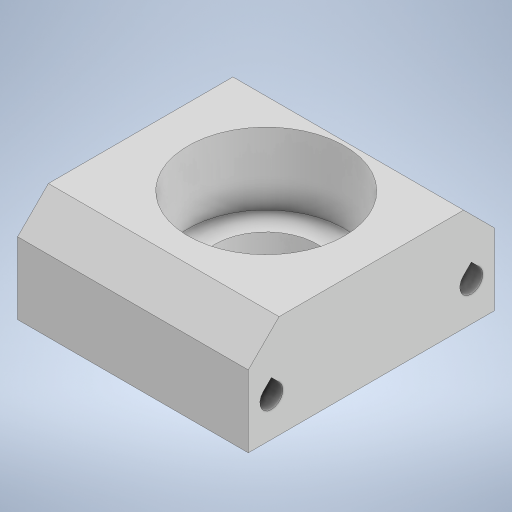
# Autodesk Inventor part: Część1-01
Saved by Autodesk Inventor 2023 (Build 270158000, 158)
## iProperties
Created: 2023-04-06
Part Number: Część1-01
Material: Ogólny
Document SubType Name: Modeling
Designer: Kamil
Density: 1 g/cm^3
Appearance: Domyślna
Author: Kamil
Autodesk Inventor part; units mm, degrees
ref_plane "YZ Plane" through (0, 0, 0) normal (1, 0, 0) x (0, 1, 0)
ref_plane "XZ Plane" through (0, 0, 0) normal (0, 1, 0) x (-1, 0, 0)
ref_plane "XY Plane" through (0, 0, 0) normal (0, 0, 1) x (1, 0, 0)
sketch "Szkic1" plane through (0, 0, 0) normal (0, 1, 0) x (-1, 0, 0)
  line L0 (22.5, 24) -> (-22.5, 24)
  line L1 (-22.5, 24) -> (-22.5, -24)
  line L2 (-22.5, -24) -> (22.5, -24)
  line L3 (22.5, -24) -> (22.5, 24)
  line L4 (22.5, 24) -> (-22.5, -24) construction
  line L5 (-22.5, 24) -> (22.5, -24) construction
  point P0 (0, 0)
  dimension "d0" = 45
  dimension "d1" = 48
  constraints: 12 end point, 2 midpoint, 2 parallel, 1 horizontal, 1 perpendicular
  measures "d0" distance of L2.end L1.end
  measures "d1" distance of L1.end L0.end
extrude "Wyciągnięcie proste1" add sketch "Szkic1" along normal blind 20
sketch "Szkic2" plane through (0, 20, 0) normal (0, 1, 0) x (1, 0, 0)
  line L0 (0, 0) -> (0, 2) construction
  dimension "d4" = 2
  constraints: 2 end point, 1 coincident, 1 vertical
  measures "d4" distance of L0.start L0.end
hole "Otwór1" at (0, 20, -2) direction (0, -1, 0) diameter 20 end through all counterbore diameter 30.5 counterbore depth 14
chamfer "Faza1" distance 6 angle 45 2 edges at (0, 20, -24) (0, 20, 24)
sketch "Szkic3" plane through (22.5, 0, 24) normal (1, 0, 0) x (0, 0, -1)
  line L0 (0, 0) -> (4.5, 0)
  line L1 (24, 0) -> (24, 9.8003)
  arc A0 (2.909, 8.891) -> (6.091, 8.891) centre (4.5, 7.3) ccw
  line L2 (4.5, 10.482) -> (6.091, 8.891)
  line L3 (4.5, 10.482) -> (2.909, 8.891)
  line L4 (0, 0) -> (48, 0) projected
  line L5 (0, 0) -> (0, 14) projected
  arc A1 (41.909, 8.891) -> (45.091, 8.891) centre (43.5, 7.3) ccw
  line L6 (43.5, 10.482) -> (41.909, 8.891)
  line L7 (43.5, 10.482) -> (45.091, 8.891)
  dimension "d17" = 4.5
  dimension "d20" = 7.3
  dimension "d21" = 4.5
  constraints: 12 end point, 4 point on circle, 4 symmetric about line, 2 centre point, 2 coincident, 1 horizontal, 1 tangent, 1 vertical, 1 other
  measures "d17" diameter of A0
  measures "d20" distance from line of L4 A0.centre
  measures "d21" distance from line of L5 A0.centre
extrude "Wyciągnięcie proste2" cut sketch "Szkic3" against normal through all
sketch "Szkic4" plane through (22.5, 0, -24) normal (0, 0, -1) x (-1, 0, 0)
  line L0 (12.305, 10.2206) -> (32.695, 10.2206) construction
  line L1 (32.695, 10.2206) -> (32.695, 3.7794) construction
  line L2 (32.695, 3.7794) -> (12.305, 3.7794) construction
  line L3 (12.305, 3.7794) -> (12.305, 10.2206) construction
  line L4 (22.5, -0.0035) -> (22.5, 22.4866) construction
  line L5 (0, 8.891) -> (45, 8.891) construction
  line L6 (0, 0) -> (0, 14) construction
  line L7 (17.4064, 4.002) -> (12.9229, 4.002)
  line L8 (12.9229, 4.002) -> (12.9229, 4.9956)
  spline S0 degree 2 poles (12.9229, 4.9956) (13.4914, 5.4503) (14.4009, 6.2511) (14.742, 6.612) knots 0 0 0 1 2 2 2
  spline S1 degree 2 poles (14.742, 6.612) (15.1919, 7.0816) (15.5923, 7.7984) (15.5923, 8.1741) knots 0 0 0 1 2 2 2
  spline S2 degree 2 poles (15.5923, 8.1741) (15.5923, 8.5992) (15.0831, 9.054) (14.6283, 9.054) knots 0 0 0 1 2 2 2
  spline S3 degree 2 poles (14.6283, 9.054) (14.396, 9.054) (13.9808, 8.9403) (13.7682, 8.8513) knots 0 0 0 1 2 2 2
  spline S4 degree 2 poles (13.7682, 8.8513) (13.5606, 8.7574) (13.264, 8.5597) (13.1898, 8.5102) knots 0 0 0 1 2 2 2
  line L9 (13.1898, 8.5102) -> (13.0712, 8.5102)
  line L10 (13.0712, 8.5102) -> (13.0712, 9.84)
  spline S5 degree 2 poles (13.0712, 9.84) (13.3282, 9.9635) (14.4257, 10.2206) (14.9348, 10.2206) knots 0 0 0 1 2 2 2
  spline S6 degree 2 poles (14.9348, 10.2206) (16.0223, 10.2206) (17.1395, 9.2517) (17.1395, 8.3768) knots 0 0 0 1 2 2 2
  spline S7 degree 2 poles (17.1395, 8.3768) (17.1395, 7.8379) (16.6304, 6.7999) (16.0421, 6.2067) knots 0 0 0 1 2 2 2
  spline S8 degree 2 poles (16.0421, 6.2067) (15.6714, 5.8409) (14.9744, 5.2724) (14.8211, 5.1537) knots 0 0 0 1 2 2 2
  line L11 (14.8211, 5.1537) -> (17.4064, 5.1537)
  line L12 (17.4064, 5.1537) -> (17.4064, 4.002)
  line L13 (23.6893, 4.002) -> (23.6893, 6.3006)
  spline S9 degree 2 poles (23.6893, 6.3006) (23.6893, 6.6417) (23.6646, 7.1063) (23.6053, 7.2546) knots 0 0 0 1 2 2 2
  spline S10 degree 2 poles (23.6053, 7.2546) (23.5411, 7.4029) (23.284, 7.5364) (23.0517, 7.5364) knots 0 0 0 1 2 2 2
  spline S11 degree 2 poles (23.0517, 7.5364) (22.8885, 7.5364) (22.5722, 7.393) (22.3843, 7.2596) knots 0 0 0 1 2 2 2
  line L14 (22.3843, 7.2596) -> (22.3843, 4.002)
  line L15 (22.3843, 4.002) -> (20.9409, 4.002)
  line L16 (20.9409, 4.002) -> (20.9409, 6.3006)
  spline S12 degree 2 poles (20.9409, 6.3006) (20.9409, 6.6367) (20.9112, 7.1063) (20.8519, 7.2546) knots 0 0 0 1 2 2 2
  spline S13 degree 2 poles (20.8519, 7.2546) (20.7876, 7.4029) (20.5306, 7.5364) (20.2983, 7.5364) knots 0 0 0 1 2 2 2
  spline S14 degree 2 poles (20.2983, 7.5364) (20.1252, 7.5364) (19.7842, 7.3733) (19.626, 7.2596) knots 0 0 0 1 2 2 2
  line L17 (19.626, 7.2596) -> (19.626, 4.002)
  line L18 (19.626, 4.002) -> (18.1924, 4.002)
  line L19 (18.1924, 4.002) -> (18.1924, 8.6041)
  line L20 (18.1924, 8.6041) -> (19.626, 8.6041)
  line L21 (19.626, 8.6041) -> (19.626, 8.095)
  spline S15 degree 2 poles (19.626, 8.095) (19.9769, 8.3916) (20.6047, 8.7277) (20.9953, 8.7277) knots 0 0 0 1 2 2 2
  spline S16 degree 2 poles (20.9953, 8.7277) (21.4154, 8.7277) (22.0581, 8.3273) (22.2261, 7.9269) knots 0 0 0 1 2 2 2
  spline S17 degree 2 poles (22.2261, 7.9269) (22.6364, 8.3125) (23.368, 8.7277) (23.7437, 8.7277) knots 0 0 0 1 2 2 2
  spline S18 degree 2 poles (23.7437, 8.7277) (24.065, 8.7277) (24.5742, 8.5251) (24.7472, 8.3174) knots 0 0 0 1 2 2 2
  spline S19 degree 2 poles (24.7472, 8.3174) (24.94, 8.095) (25.1328, 7.487) (25.1328, 6.9976) knots 0 0 0 1 2 2 2
  line L22 (25.1328, 6.9976) -> (25.1328, 4.002)
  line L23 (25.1328, 4.002) -> (23.6893, 4.002)
  line L24 (31.6876, 4.002) -> (31.6876, 6.3006)
  spline S20 degree 2 poles (31.6876, 6.3006) (31.6876, 6.6417) (31.6628, 7.1063) (31.6035, 7.2546) knots 0 0 0 1 2 2 2
  spline S21 degree 2 poles (31.6035, 7.2546) (31.5393, 7.4029) (31.2822, 7.5364) (31.0499, 7.5364) knots 0 0 0 1 2 2 2
  spline S22 degree 2 poles (31.0499, 7.5364) (30.8868, 7.5364) (30.5704, 7.393) (30.3825, 7.2596) knots 0 0 0 1 2 2 2
  line L25 (30.3825, 7.2596) -> (30.3825, 4.002)
  line L26 (30.3825, 4.002) -> (28.9391, 4.002)
  line L27 (28.9391, 4.002) -> (28.9391, 6.3006)
  spline S23 degree 2 poles (28.9391, 6.3006) (28.9391, 6.6367) (28.9094, 7.1063) (28.8501, 7.2546) knots 0 0 0 1 2 2 2
  spline S24 degree 2 poles (28.8501, 7.2546) (28.7859, 7.4029) (28.5288, 7.5364) (28.2965, 7.5364) knots 0 0 0 1 2 2 2
  spline S25 degree 2 poles (28.2965, 7.5364) (28.1235, 7.5364) (27.7824, 7.3733) (27.6242, 7.2596) knots 0 0 0 1 2 2 2
  line L28 (27.6242, 7.2596) -> (27.6242, 4.002)
  line L29 (27.6242, 4.002) -> (26.1906, 4.002)
  line L30 (26.1906, 4.002) -> (26.1906, 8.6041)
  line L31 (26.1906, 8.6041) -> (27.6242, 8.6041)
  line L32 (27.6242, 8.6041) -> (27.6242, 8.095)
  spline S26 degree 2 poles (27.6242, 8.095) (27.9752, 8.3916) (28.603, 8.7277) (28.9935, 8.7277) knots 0 0 0 1 2 2 2
  spline S27 degree 2 poles (28.9935, 8.7277) (29.4137, 8.7277) (30.0563, 8.3273) (30.2244, 7.9269) knots 0 0 0 1 2 2 2
  spline S28 degree 2 poles (30.2244, 7.9269) (30.6346, 8.3125) (31.3663, 8.7277) (31.7419, 8.7277) knots 0 0 0 1 2 2 2
  spline S29 degree 2 poles (31.7419, 8.7277) (32.0633, 8.7277) (32.5724, 8.5251) (32.7454, 8.3174) knots 0 0 0 1 2 2 2
  spline S30 degree 2 poles (32.7454, 8.3174) (32.9382, 8.095) (33.131, 7.487) (33.131, 6.9976) knots 0 0 0 1 2 2 2
  line L33 (33.131, 6.9976) -> (33.131, 4.002)
  line L34 (33.131, 4.002) -> (31.6876, 4.002)
  point P0 (22.5, 0)
  point P1 (22.5, 10.2206)
  point P2 (22.5, 8.891)
  point P3 (32.695, 7)
  point P4 (0, 7)
  constraints: 4 midpoint, 2 end point, 1 horizontal alignment, 1 vertical, 1 vertical alignment, 2 other
extrude "Wyciągnięcie proste3" cut sketch "Szkic4" against normal blind 0.5
